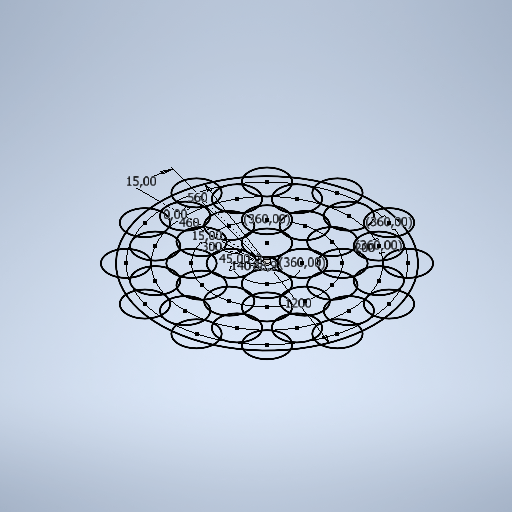
# Autodesk Inventor part: 000 DIM PNS-Filter column D1200
Saved by Autodesk Inventor 2025 (Build 290162010, 162A)
## iProperties
Created: 2025-02-12
Part Number: 000 DIM PNS-Filter column D1200
Material: Generic
Document SubType Name: Modeling
Designer: pokla
Density: 1 g/cm^3
Appearance: Default
MAIN_filter_diam: 1200,000 mm
MAIN_hight: 2450.000 mm
Accsess_hatch_diameter: 530,000 mm
Accsess_hatch_lenght: 120,000 mm
Charging_hatch_width: 400,000 mm
Charging_hatch_hight: 180,000 mm
Charging_hatch_lenght: 120,000 mm
Author: pokla
Autodesk Inventor part; units mm, degrees
ref_plane "YZ Plane" through (0, 0, 0) normal (1, 0, 0) x (0, 1, 0)
ref_plane "XZ Plane" through (0, 0, 0) normal (0, 1, 0) x (-1, 0, 0)
ref_plane "XY Plane" through (0, 0, 0) normal (0, 0, 1) x (1, 0, 0)
sketch "Sketch1" plane through (0, 0, 0) normal (0, 0, 1) x (1, 0, 0)
  circle A0 centre (0, 0) radius 44.45
  circle A1 centre (0, 0) radius 41.45
  circle A2 centre (0, 0) radius 600
  circle A3 centre (144.9387, 540.9185) radius 100
  circle A4 centre (-144.9387, 540.9185) radius 100
  circle A5 centre (-395.9798, 395.9798) radius 100
  circle A6 centre (-540.9185, 144.9387) radius 100
  circle A7 centre (-540.9185, -144.9387) radius 100
  circle A8 centre (-395.9798, -395.9798) radius 100
  circle A9 centre (-144.9387, -540.9185) radius 100
  circle A10 centre (144.9387, -540.9185) radius 100
  circle A11 centre (395.9798, -395.9798) radius 100
  circle A12 centre (540.9185, -144.9387) radius 100
  circle A13 centre (230, 398.3717) radius 100
  circle A14 centre (0, 460) radius 100
  circle A15 centre (-230, 398.3717) radius 100
  circle A16 centre (-398.3717, 230) radius 100
  circle A17 centre (-460, 0) radius 100
  circle A18 centre (-398.3717, -230) radius 100
  circle A19 centre (-230, -398.3717) radius 100
  circle A20 centre (0, -460) radius 100
  circle A21 centre (230, -398.3717) radius 100
  circle A22 centre (398.3717, -230) radius 100
  circle A23 centre (-212.132, 212.132) radius 100
  circle A24 centre (-289.7777, 77.6457) radius 100
  circle A25 centre (-289.7777, -77.6457) radius 100
  circle A26 centre (-212.132, -212.132) radius 100
  circle A27 centre (-77.6457, -289.7777) radius 100
  circle A28 centre (77.6457, -289.7777) radius 100
  circle A29 centre (212.132, -212.132) radius 100
  circle A30 centre (289.7777, -77.6457) radius 100
  circle A31 centre (98.9949, 98.9949) radius 100
  circle A32 centre (289.7777, 77.6457) radius 100
  circle A33 centre (212.132, 212.132) radius 100
  circle A34 centre (-98.9949, 98.9949) radius 100
  circle A35 centre (-98.9949, -98.9949) radius 100
  circle A36 centre (98.9949, -98.9949) radius 100
  circle A37 centre (460, 0) radius 100
  circle A38 centre (398.3717, 230) radius 100
  circle A39 centre (77.6457, 289.7777) radius 100
  circle A40 centre (-77.6457, 289.7777) radius 100
  circle A41 centre (540.9185, 144.9387) radius 100
  circle A42 centre (395.9798, 395.9798) radius 100
  line L0 (0, 0) -> (-600, 0) construction
  line L1 (0, 0) -> (-540.9185, 144.9387) construction
  line L2 (-460, 0) -> (0, 0) construction
  line L3 (0, 0) -> (-289.7777, -77.6457) construction
  line L4 (-98.9949, -98.9949) -> (0, 0) construction
  dimension "d2" = 1200
  dimension "d0" = 88.9
  dimension "d1" = 3
  dimension "d5" = 360
  dimension "d9" = 360
  dimension "d11" = 200
  dimension "d14" = 360
  dimension "d18" = 360
  dimension "d20" = 15
  dimension "d21" = 0
  dimension "d22" = 15
  dimension "d23" = 45
  dimension "d24" = 140
  dimension "d25" = 300
  dimension "d26" = 460
  dimension "d27" = 560
  constraints: 42 centre point, 10 end point, 3 equal radius, 2 coincident, 1 horizontal, 1 horizontal alignment, 86 other
  measures "d0" diameter of A0
  measures "d1" radial gap between concentric circles of A0 A1
  measures "d11" diameter of A13
  measures "d20" angle of L0 L1
  measures "d21" distance between parallel lines of L0 L2
  measures "d22" angle of L3 L2
  measures "d23" angle of L4 L2
  measures "d24" distance of L4.start L0.start
  measures "d25" distance of L0.start L3.end
  measures "d26" distance of L2.start L0.start
  measures "d27" distance of L0.start L1.end
sketch "Sketch2" plane through (0, 0, 0) normal (0, 0, 1) x (1, 0, 0)
  point P0 (0, 0)
  point P1 (-98.9949, -98.9949)
  point P2 (98.9949, -98.9949)
  point P3 (98.9949, 98.9949)
  point P4 (-98.9949, 98.9949)
  point P5 (-77.6457, 289.7777)
  point P6 (77.6457, 289.7777)
  point P7 (212.132, 212.132)
  point P8 (289.7777, 77.6457)
  point P9 (289.7777, -77.6457)
  point P10 (212.132, -212.132)
  point P11 (77.6457, -289.7777)
  point P12 (-77.6457, -289.7777)
  point P13 (0, -460)
  point P14 (230, -398.3717)
  point P15 (144.9387, -540.9185)
  point P16 (395.9798, -395.9798)
  point P17 (398.3717, -230)
  point P18 (540.9185, -144.9387)
  point P19 (460, 0)
  point P20 (540.9185, 144.9387)
  point P21 (398.3717, 230)
  point P22 (395.9798, 395.9798)
  point P23 (230, 398.3717)
  point P24 (144.9387, 540.9185)
  point P25 (0, 460)
  point P26 (-144.9387, 540.9185)
  point P27 (-230, 398.3717)
  point P28 (-212.132, 212.132)
  point P29 (-289.7777, 77.6457)
  point P30 (-289.7777, -77.6457)
  point P31 (-212.132, -212.132)
  point P32 (-398.3717, 230)
  point P33 (-395.9798, 395.9798)
  point P34 (-540.9185, 144.9387)
  point P35 (-460, 0)
  point P36 (-540.9185, -144.9387)
  point P37 (-398.3717, -230)
  point P38 (-395.9798, -395.9798)
  point P39 (-230, -398.3717)
  point P40 (-144.9387, -540.9185)
sketch "Sketch3" plane through (0, 0, 0) normal (0, 0, 1) x (1, 0, 0)
  circle A0 centre (0, 0) radius 15
  dimension "d28" = 30
  constraints: 1 centre point, 1 coincident
  measures "d28" diameter of A0
extrude "Extrusion1" add sketch "Sketch3" along normal blind 10
equation "\"MAIN_filter_diam\" = 1200"
equation "\"MAIN_hight\" = 2450"
equation "\"Accsess_hatch_lenght\" = 120"
equation "\"Accsess_hatch_diameter\" = 530"
equation "\"Charging_hatch_width\" = 400"
equation "\"Charging_hatch_hight\" = 180"
equation "\"Charging_hatch_lenght\" = 120"
body "Solid1"
